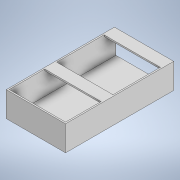
# Autodesk Inventor part: ShootingMech_Housing
Saved by Autodesk Inventor 2020 (Build 240168000, 168)
## iProperties
Created: 2021-12-08
Part Number: ShootingMech_Housing
Material: Generic
Document SubType Name: Modeling
Designer: danie
Density: 1 g/cm^3
Appearance: Default
Author: danie
Autodesk Inventor part; units mm, degrees
ref_plane "YZ Plane" through (0, 0, 0) normal (1, 0, 0) x (0, 1, 0)
ref_plane "XZ Plane" through (0, 0, 0) normal (0, 1, 0) x (-1, 0, 0)
ref_plane "XY Plane" through (0, 0, 0) normal (0, 0, 1) x (1, 0, 0)
sketch "Sketch1" plane through (0, 0, 0) normal (0, 1, 0) x (-1, 0, 0)
  line L0 (0, 0) -> (-127, 0)
  line L1 (-127, 0) -> (-127, 228.6)
  line L2 (-127, 228.6) -> (0, 228.6)
  line L3 (0, 228.6) -> (0, 0)
  dimension "d0" = 127
  dimension "d1" = 228.6
  constraints: 8 end point, 2 parallel, 1 horizontal, 1 perpendicular
  measures "d0" distance of L1.end L2.end
  measures "d1" distance of L0.end L1.end
extrude "Extrusion1" add sketch "Sketch1" along normal blind 3.175
sketch "Sketch2" plane through (0, 3.175, 0) normal (0, 1, 0) x (1, 0, 0)
  line L0 (0, 0) -> (0, -228.6) projected
  line L1 (0, 0) -> (3.175, 0)
  line L2 (3.175, 0) -> (3.175, -228.6)
  line L3 (3.175, -228.6) -> (0, -228.6)
  line L4 (0, -228.6) -> (0, 0)
  dimension "d4" = 3.175
  dimension "d5" = 228.6
  constraints: 8 end point, 2 parallel, 1 horizontal, 1 perpendicular
  measures "d4" distance of L2.end L3.end
  measures "d5" distance of L1.end L2.end
extrude "Extrusion2" add sketch "Sketch2" along normal blind 50.8
sketch "Sketch3" plane through (0, 3.175, 0) normal (0, 1, 0) x (1, 0, 0)
  line L0 (127, -228.6) -> (127, 0) projected
  line L1 (127, 0) -> (123.825, 0)
  line L2 (123.825, 0) -> (123.825, -228.6)
  line L3 (123.825, -228.6) -> (127, -228.6)
  line L4 (127, -228.6) -> (127, 0)
  point P0 (0, 0)
  dimension "d8" = 3.175
  dimension "d9" = 228.6
  constraints: 8 end point, 2 parallel, 1 horizontal, 1 perpendicular
  measures "d8" distance of L3.end L2.end
  measures "d9" distance of L2.end L1.end
extrude "Extrusion3" add sketch "Sketch3" along normal blind 50.8
sketch "Sketch6" plane through (0, 0, 228.6) normal (0, 0, 1) x (1, 0, 0)
  line L0 (0, 0) -> (127, 0) projected
  line L1 (0, 53.975) -> (127, 53.975)
  line L2 (127, 53.975) -> (127, 0)
  line L3 (127, 0) -> (0, 0)
  line L4 (0, 0) -> (0, 53.975)
  constraints: 8 end point, 2 parallel, 1 horizontal, 1 perpendicular
extrude "Extrusion4" add sketch "Sketch6" along normal blind 3.175
sketch "Sketch7" plane through (3.175, 3.175, 0) normal (1, 0, 0) x (0, 0, -1)
  line L0 (-228.6, 50.8) -> (-152.4, 50.8) construction
  line L1 (0, 50.8) -> (-231.775, 50.8) construction
  line L2 (-228.6, 50.8) -> (-152.4, 50.8) construction
  line L3 (-152.4, 50.8) -> (-127, 50.8)
  line L4 (-127, 50.8) -> (-127, 47.625)
  line L5 (-127, 47.625) -> (-152.4, 47.625)
  line L6 (-152.4, 47.625) -> (-152.4, 50.8)
  point P0 (0, -3.175)
  dimension "d19" = 76.2
  dimension "d20" = 0
  dimension "d21" = 25.4
  dimension "d22" = 3.175
  constraints: 12 end point, 2 collinear, 2 horizontal, 2 parallel, 1 perpendicular
  measures "d19" distance of L0.start L0.end
  measures "d20" distance between parallel lines of L0 L2
  measures "d21" distance of L4.end L5.end
  measures "d22" distance of L3.end L4.end
extrude "Extrusion5" add sketch "Sketch7" along normal blind 120.65
sketch "Sketch8" plane through (0, 53.975, 0) normal (0, 1, 0) x (1, 0, 0)
  line L0 (3.175, -127) -> (3.175, 0) projected
  line L1 (3.175, 0) -> (123.825, 0)
  line L2 (123.825, 0) -> (123.825, -25.4)
  line L3 (123.825, -25.4) -> (3.175, -25.4)
  line L4 (3.175, -25.4) -> (3.175, 0)
  point P0 (0, 0)
  point P1 (3.175, -25.4)
  dimension "d25" = 120.65
  dimension "d26" = 25.4
  constraints: 8 end point, 2 parallel, 1 horizontal, 1 perpendicular
  measures "d25" distance of L2.end L3.end
  measures "d26" distance of L1.end L2.end
extrude "Extrusion6" add sketch "Sketch8" against normal blind 3.175
body "Solid1"
